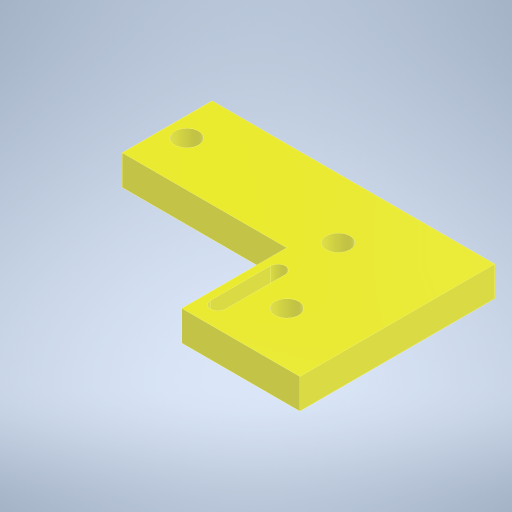
# Autodesk Inventor part: креп_опт
Saved by Autodesk Inventor 2023.1 (Build 271208000, 208)
## iProperties
Created: 2025-12-30
Part Number: креп_опт
Material: Полипропилен
Document SubType Name: Modeling
Designer: DELL
Density: 0.899 g/cm^3
Appearance: Желтый
Author: DELL
Autodesk Inventor part; units mm, degrees
ref_plane "YZ Plane" through (0, 0, 0) normal (1, 0, 0) x (0, 1, 0)
ref_plane "XZ Plane" through (0, 0, 0) normal (0, 1, 0) x (-1, 0, 0)
ref_plane "XY Plane" through (0, 0, 0) normal (0, 0, 1) x (1, 0, 0)
sketch "Эскиз9" plane through (0, 0, 0) normal (0, 1, 0) x (-1, 0, 0)
  line L0 (-7.875, 7) -> (7.875, 7)
  line L1 (7.875, 7) -> (7.875, -7)
  line L2 (7.875, -7) -> (-7.875, -7)
  line L3 (-7.875, -7) -> (-7.875, 7)
  line L4 (-7.875, 7) -> (7.875, -7) construction
  line L5 (7.875, 7) -> (-7.875, -7) construction
  circle A0 centre (0.875, 0) radius 1.6
  point P0 (0, 0)
  point P1 (7.875, 0)
  dimension "d56" = 15.75
  dimension "d57" = 14
  dimension "d58" = 3.2
  dimension "d74" = 7
  constraints: 12 end point, 3 midpoint, 2 parallel, 1 centre point, 1 horizontal, 1 perpendicular
  measures "d56" distance of L1.end L2.end
  measures "d57" distance of L0.end L1.end
  measures "d58" diameter of A0
  measures "d74" distance of point (7.875, 0) A0.centre
extrude "Выдавливание9" add sketch "Эскиз9" along normal blind 4
sketch "Эскиз10" plane through (0, 4, 0) normal (0, 1, 0) x (1, 0, 0)
  line L0 (7.875, 19) -> (-29.825, 19)
  line L1 (-29.825, 19) -> (-29.825, 7)
  line L2 (-29.825, 7) -> (7.875, 7)
  line L3 (7.875, 7) -> (7.875, 19)
  line L4 (7.875, 19) -> (-29.825, 7) construction
  line L5 (-29.825, 19) -> (7.875, 7) construction
  line L6 (7.875, 7) -> (-7.875, 7) projected
  line L7 (-7.875, 7) -> (-7.875, -7) projected
  line L8 (7.875, -7) -> (7.875, 7) projected
  point P0 (0, 0)
  point P1 (-10.975, 13)
  point P2 (0, 7)
  point P3 (7.875, 13)
  dimension "d71" = 37.7
  dimension "d72" = 12
  constraints: 12 end point, 4 midpoint, 2 parallel, 2 point on line, 1 horizontal, 1 perpendicular
  measures "d71" distance of L2.end L1.end
  measures "d72" distance of L1.end L0.end
extrude "Выдавливание10" add sketch "Эскиз10" against normal blind 4
sketch "Эскиз11" plane through (0, 4, 0) normal (0, 1, 0) x (1, 0, 0)
  circle A0 centre (-14.5, 13) radius 1.6 construction
  circle A1 centre (7.7, 11) radius 1.6 construction
  circle A2 centre (-27.225, 13) radius 1.6
  line L0 (-29.825, 19) -> (-29.825, 7) projected
  line L1 (-29.825, 7) -> (-7.875, 7) projected
  circle A3 centre (-5.025, 11) radius 1.6
  line L2 (7.875, -7) -> (7.875, 19) projected
  point P0 (-29.825, 13)
  dimension "d75" = 3.2
  dimension "d76" = 2.6
  dimension "d77" = 6
  dimension "d78" = 3.2
  dimension "d79" = 4
  dimension "d80" = 12.9
  constraints: 2 centre point, 1 midpoint
  measures "d75" diameter of A2
  measures "d76" distance of point (-29.825, 13) A2.centre
  measures "d77" distance from line of L1 A2.centre
  measures "d78" diameter of A3
  measures "d79" distance from line of L1 A3.centre
  measures "d80" distance from line of L2 A3.centre
extrude "Выдавливание11" cut sketch "Эскиз11" against normal blind 4
sketch "Эскиз12" plane through (0, 4, 0) normal (0, 1, 0) x (1, 0, 0)
  line L0 (-5.875, 4.8221) -> (-5.875, -5.1779) construction
  line L1 (-6.875, 3.8221) -> (-6.875, -4.1779)
  line L2 (-4.875, -4.1779) -> (-4.875, 3.8221)
  arc A0 (-4.875, 3.8221) -> (-6.875, 3.8221) centre (-5.875, 3.8221) ccw
  arc A1 (-6.875, -4.1779) -> (-4.875, -4.1779) centre (-5.875, -4.1779) ccw
  circle A2 centre (-0.875, 0) radius 1.6 projected
  point P0 (0, 0)
  point P1 (-5.875, -0.1779)
  dimension "d81" = 10
  dimension "d82" = 2
  dimension "d83" = 5
  constraints: 8 end point, 6 point on circle, 4 tangent, 2 centre point, 2 point on line, 1 midpoint, 1 parallel, 1 vertical
  measures "d81" distance of L0.start L0.end
  measures "d82" diameter of A1
  measures "d83" distance from line of A2.centre L0
extrude "Выдавливание12" cut sketch "Эскиз12" against normal blind 4
